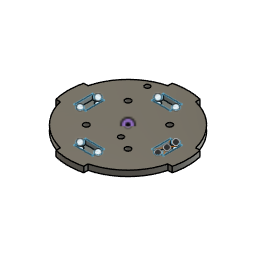
Button Plate (Autodesk Fusion 360 design; units mm, degrees)
Autodesk Fusion 360 part; units mm, degrees
note: some values were not read from the file. Set by a fixed rule: which sketch regions a step uses.
sketch "Plate" plane through (0, 0, 0) normal (0, 1, 0) x (1, 0, 0)
  circle A0 centre (0, 0) radius 21.5
  circle A1 centre (0, 0) radius 20
  line L0 (5, -23) -> (-5, -23)
  line L1 (-5, -23) -> (-5, 23)
  line L2 (-5, 23) -> (5, 23)
  line L3 (5, 23) -> (5, -23)
  line L4 (23, -5) -> (-23, -5)
  line L5 (-23, -5) -> (-23, 5)
  line L6 (-23, 5) -> (23, 5)
  line L7 (23, 5) -> (23, -5)
  line L8 (7.5, -7.5) -> (-7.5, -7.5) construction
  line L9 (-7.5, -7.5) -> (-7.5, 7.5) construction
  line L10 (-7.5, 7.5) -> (7.5, 7.5) construction
  line L11 (7.5, 7.5) -> (7.5, -7.5) construction
  line L12 (7.5, -7.5) -> (-7.5, 7.5) construction
  line L13 (-7.5, -7.5) -> (7.5, 7.5) construction
  circle A2 centre (7.5, 7.5) radius 1
  circle A3 centre (7.5, -7.5) radius 1
  circle A4 centre (-7.5, -7.5) radius 1
  circle A5 centre (-7.5, 7.5) radius 1
  circle A6 centre (2.5, -5) radius 0.9
  circle A7 centre (-8.5, 15.5) radius 0.9
  dimension "d1" = 43
  dimension "d2" = 40
  dimension "d3" = 10
  dimension "d4" = 46
  dimension "d5" = 10
  dimension "d6" = 15
  dimension "d7" = 15
  dimension "d8" = 2
  dimension "d9" = 2
  dimension "d10" = 2
  dimension "d11" = 2
  dimension "d12" = 1.8
  dimension "d13" = 1.8
  constraint coincident A0.centre A1.centre
  constraint horizontal L0
  constraint perpendicular L0 L1
  constraint parallel L0 L2
  constraint parallel L1 L3
  constraint horizontal L4
  constraint perpendicular L4 L5
  constraint parallel L4 L6
  constraint parallel L5 L7
  constraint horizontal L8
  constraint perpendicular L8 L9
  constraint parallel L8 L10
  constraint parallel L9 L11
  constraint coincident L12 A0.centre
  constraint coincident L13 A0.centre
  constraint coincident L10.end L11.start
  constraint coincident L8.start L11.end
  constraint coincident L8.end L9.start
  constraint coincident L9.end L10.start
  measures "d1" diameter of A0
  measures "d2" diameter of A1
  measures "d3" distance of L1.end L2.end
  measures "d4" distance of L5.end L6.end
  measures "d5" distance of L4.end L5.end
  measures "d6" distance of L9.end L10.end
  measures "d7" distance of L8.end L9.end
  measures "d8" diameter of A2
  measures "d9" diameter of A3
  measures "d10" diameter of A4
  measures "d11" diameter of A5
  measures "d12" diameter of A6
  measures "d13" diameter of A7
extrude "Extrude1" add sketch "Plate" against normal blind 2 contours A0 A1 L4 L6 | A0 A1 L1 L3 | A1 L3 L6 | A1 L3 L4 L6 | A0 A1 L1 L3 | A1 L3 L4 | A1 L1 L3 L6 | L1 L3 L4 L6 A6 | A1 L1 L3 L4 A6 | A0 A1 L4 L6 | A1 L1 L6 | A1 L1 L4 L6 | A1 L1 L4
sketch "Buttons" plane through (0, 0, 0) normal (0, 1, 0) x (1, 0, 0)
  line L0 (16, -3.25) -> (12, -3.25)
  line L1 (12, -3.25) -> (12, 3.25)
  line L2 (12, 3.25) -> (16, 3.25)
  line L3 (16, 3.25) -> (16, -3.25)
  line L4 (16, -3.25) -> (12, 3.25) construction
  line L5 (12, -3.25) -> (16, 3.25) construction
  circle A0 centre (14, 3.25) radius 1
  circle A1 centre (14, -3.25) radius 1
  circle A2 centre (-3.25, 14) radius 1
  circle A3 centre (3.25, 14) radius 1
  line L6 (3.25, 12) -> (-3.25, 12)
  line L7 (-3.25, 12) -> (-3.25, 16)
  line L8 (3.25, 16) -> (3.25, 12)
  line L9 (-3.25, 16) -> (3.25, 16)
  circle A4 centre (-14, -3.25) radius 1
  circle A5 centre (-14, 3.25) radius 1
  line L10 (-12, 3.25) -> (-12, -3.25)
  line L11 (-12, -3.25) -> (-16, -3.25)
  line L12 (-16, 3.25) -> (-12, 3.25)
  line L13 (-16, -3.25) -> (-16, 3.25)
  circle A6 centre (3.25, -14) radius 1
  circle A7 centre (-3.25, -14) radius 1
  line L14 (-3.25, -12) -> (3.25, -12)
  line L15 (3.25, -12) -> (3.25, -16)
  line L16 (-3.25, -16) -> (-3.25, -12)
  line L17 (3.25, -16) -> (-3.25, -16)
  point P0 (14, 0)
  dimension "d16" = 4
  dimension "d17" = 6.5
  dimension "d18" = 2
  dimension "d19" = 2
  dimension "d21" = 360
  constraint horizontal L0
  constraint perpendicular L0 L1
  constraint parallel L0 L2
  constraint parallel L1 L3
  constraint coincident L4 P0
  constraint coincident L5 P0
  constraint midpoint L2 A0.centre
  constraint midpoint L0 A1.centre
  measures "d16" distance of L1.end L2.end
  measures "d17" distance of L0.end L1.end
  measures "d18" diameter of A0
  measures "d19" diameter of A1
extrude "Extrude2" cut sketch "Buttons" against normal blind 1.8 contours L0 L1 L2 L3 A0 A1 | A2 A3 L6 L7 L8 L9 | A4 A5 L10 L11 L12 L13 | A6 A7 L14 L15 L16 L17
extrude "Extrude3" cut sketch "Buttons" against normal blind 3 contours L0 A1 | L0 A1 | L2 A0 | L2 A0 | A2 L7 | A2 L7 | A3 L8 | A3 L8 | A4 L11 | A4 L11 | A5 L12 | A5 L12 | A6 L15 | A6 L15 | A7 L16 | A7 L16
named bodies: "Button Plate"
